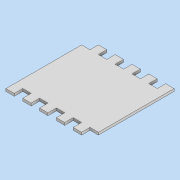
# Autodesk Inventor part: simple wall test
Saved by Autodesk Inventor 2020 (Build 240168000, 168)
## iProperties
Created: 2020-12-17
Part Number: simple wall test
Material: Generic
Document SubType Name: Modeling
Designer: solar
Density: 1 g/cm^3
Appearance: Default
Author: solar
Autodesk Inventor part; units mm, degrees
ref_plane "YZ Plane" through (0, 0, 0) normal (1, 0, 0) x (0, 1, 0)
ref_plane "XZ Plane" through (0, 0, 0) normal (0, 1, 0) x (-1, 0, 0)
ref_plane "XY Plane" through (0, 0, 0) normal (0, 0, 1) x (1, 0, 0)
sketch "Sketch1" plane through (0, 0, 0) normal (0, 1, 0) x (-1, 0, 0)
  line L0 (-100, 80) -> (-100, -100)
  line L1 (100, -80) -> (100, 100)
  line L2 (100, 100) -> (-100, -100) construction
  line L3 (-100, 100) -> (100, -100) construction
  line L4 (100, -80) -> (80, -80)
  line L5 (80, -80) -> (80, -100)
  line L6 (80, -100) -> (60, -100)
  line L7 (60, -100) -> (60, -80)
  line L8 (60, -80) -> (40, -80)
  line L9 (40, -80) -> (40, -100)
  line L10 (40, -100) -> (20, -100)
  line L11 (20, -100) -> (20, -80)
  line L12 (20, -80) -> (0, -80)
  line L13 (0, -80) -> (0, -100)
  line L14 (0, -100) -> (-20, -100)
  line L15 (-20, -100) -> (-20, -80)
  line L16 (-20, -80) -> (-40, -80)
  line L17 (-40, -80) -> (-40, -100)
  line L18 (-40, -100) -> (-60, -100)
  line L19 (-60, -100) -> (-60, -80)
  line L20 (-60, -80) -> (-80, -80)
  line L21 (-80, -80) -> (-80, -100)
  line L22 (-100, -100) -> (-80, -100)
  line L23 (-60, -100) -> (-40, -100)
  line L24 (-20, -100) -> (0, -100)
  line L25 (20, -100) -> (40, -100)
  line L26 (60, -100) -> (80, -100)
  line L27 (80, 100) -> (80, 80)
  line L28 (80, 80) -> (60, 80)
  line L29 (60, 80) -> (60, 100)
  line L30 (40, 100) -> (40, 80)
  line L31 (40, 80) -> (20, 80)
  line L32 (20, 80) -> (20, 100)
  line L33 (0, 100) -> (0, 80)
  line L34 (0, 80) -> (-20, 80)
  line L35 (-20, 80) -> (-20, 100)
  line L36 (-40, 100) -> (-40, 80)
  line L37 (-40, 80) -> (-60, 80)
  line L38 (-60, 80) -> (-60, 100)
  line L39 (-80, 100) -> (-80, 80)
  line L40 (-100, 80) -> (-80, 80)
  line L41 (100, 100) -> (80, 100)
  line L42 (60, 100) -> (40, 100)
  line L43 (20, 100) -> (0, 100)
  line L44 (-20, 100) -> (-40, 100)
  line L45 (-60, 100) -> (-80, 100)
  point P0 (0, 0)
  dimension "d0" = 200
  dimension "d1" = 200
  dimension "d2" = 20
  dimension "d4" = 20
  dimension "d5" = 20
  dimension "d6" = 20
  dimension "d7" = 20
  dimension "d8" = 20
  dimension "d9" = 20
  dimension "d10" = 20
  dimension "d11" = 20
  dimension "d12" = 20
  dimension "d13" = 20
  dimension "d14" = 20
  dimension "d15" = 20
  dimension "d16" = 20
  dimension "d17" = 20
  dimension "d18" = 20
  dimension "d19" = 20
  constraints: 92 end point, 52 perpendicular, 26 parallel, 9 point on line, 5 horizontal, 2 midpoint, 2 vertical
  measures "d0" distance of L3.end L0.end
  measures "d1" distance of L0.end L3.start
  measures "d2" distance of L1.start L3.end
  measures "d4" distance of L5.end L6.end
  measures "d5" distance of L6.end L7.end
  measures "d6" distance of L7.end L8.end
  measures "d7" distance of L8.end L9.end
  measures "d8" distance of L9.end L10.end
  measures "d9" distance of L10.end L11.end
  measures "d10" distance of L11.end L12.end
  measures "d11" distance of L13.end L14.end
  measures "d12" distance of L14.end L15.end
  measures "d13" distance of L15.end L16.end
  measures "d14" distance of L16.end L17.end
  measures "d15" distance of L17.end L18.end
  measures "d16" distance of L18.end L19.end
  measures "d17" distance of L19.end L20.end
  measures "d18" distance of L27.start L27.end
  measures "d19" distance of L27.end L28.end
extrude "Extrusion1" add sketch "Sketch1" along normal blind 6
body "Solid1"
